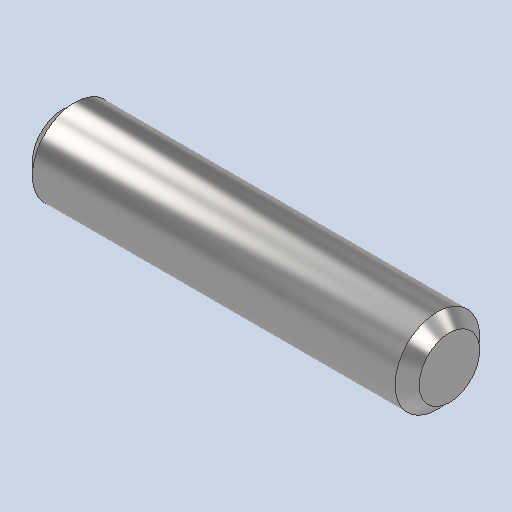
# Autodesk Inventor part: Stub
Saved by Autodesk Inventor 2023.2 (Build 272271030, 271C)
## iProperties
Created: 2023-03-23
Part Number: Stub
Material: Steel, Carbon
Document SubType Name: Modeling
Designer: Luis Valente
Density: 7.85 g/cm^3
Appearance: Semi-Polished
Author: Luis Valente
Autodesk Inventor part; units mm, degrees
ref_plane "YZ Plane" through (0, 0, 0) normal (1, 0, 0) x (0, 1, 0)
ref_plane "XZ Plane" through (0, 0, 0) normal (0, 1, 0) x (-1, 0, 0)
ref_plane "XY Plane" through (0, 0, 0) normal (0, 0, 1) x (1, 0, 0)
sketch "Sketch1" plane through (0, 0, 0) normal (1, 0, 0) x (0, 1, 0)
  circle A0 centre (0, 0) radius 7
  dimension "d0" = 14
  constraints: 1 centre point, 1 coincident
  measures "d0" diameter of A0
extrude "Extrusion1" add sketch "Sketch1" along normal blind 64
chamfer "Chamfer1" distance 2 angle 45 1 edges at (64, -7, 0) measured on face at (64, -0.8274, 0.9129)
chamfer "Chamfer2" distance 2 angle 45 1 edges at (0, -7, 0) measured on face at (0, -0.8274, 0.9129)
body "Solid1"
